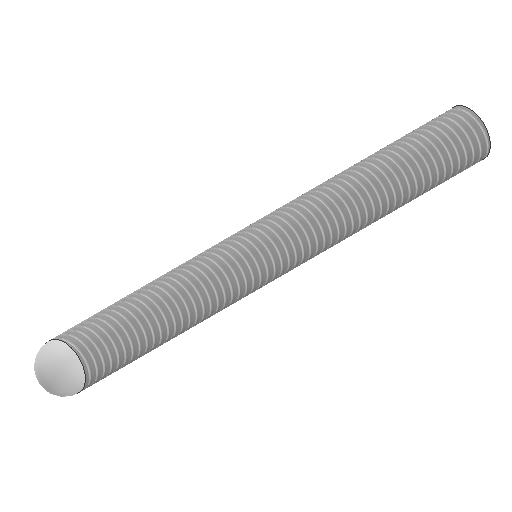
# Autodesk Inventor part: 00_Screw_Ball_Spring_Head_M3x30mm
Saved by Autodesk Inventor 2022 (Build 260153000, 153)
## iProperties
Created: 2022-09-25
Part Number: 00_Screw_Ball_Spring_Head_M3x30mm
Material: Generisch
Document SubType Name: Modeling
Designer: UC2
Density: 1 g/cm^3
Appearance: Vorgabe
Catalog Web Link: https://detail.tmall.com/item_o.htm?id=649056091807&spm=a1z09.2.0.0.366c2e8dELQBXu&_u=d1hhfjuv61c4
Vendor: Taobao
Author: UC2
Autodesk Inventor part; units mm, degrees
ref_plane "YZ Plane" through (0, 0, 0) normal (1, 0, 0) x (0, 1, 0)
ref_plane "XZ Plane" through (0, 0, 0) normal (0, 1, 0) x (-1, 0, 0)
ref_plane "XY Plane" through (0, 0, 0) normal (0, 0, 1) x (1, 0, 0)
sketch "Skizze1" plane through (0, 0, 0) normal (0, 0, 1) x (1, 0, 0)
  circle A0 centre (0, 0) radius 1.5
  dimension "d0" = 3
  constraints: 1 centre point, 1 coincident
  measures "d0" diameter of A0
extrude "Extrusion1" add sketch "Skizze1" along normal blind 30
fillet "Rundung1" radius 1.5 1 edges at (-1.5, 0, 30)
thread "Gewinde1" size "M3x0.5" class "6g" standard "ANSI Metric M Profile" full length
